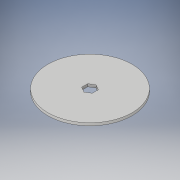
# Autodesk Inventor part: 4in Wheel Plate-ver1-1111-2019
Saved by Autodesk Inventor 2018 (Build 220112000, 112)
## iProperties
Created: 2020-01-18
Part Number: 4in Wheel Plate-ver1-1111-2019
Material: Generic
Document SubType Name: Modeling
Designer: JMHal
Density: 1 g/cm^3
Appearance: Default
Author: JMHal
Autodesk Inventor part; units mm, degrees
ref_plane "YZ Plane" through (0, 0, 0) normal (1, 0, 0) x (0, 1, 0)
ref_plane "XZ Plane" through (0, 0, 0) normal (0, 1, 0) x (-1, 0, 0)
ref_plane "XY Plane" through (0, 0, 0) normal (0, 0, 1) x (1, 0, 0)
sketch "Sketch1" plane through (0, 0, 0) normal (0, 1, 0) x (-1, 0, 0)
  circle A0 centre (0, 0) radius 50.8
  dimension "d0" = 101.6
  constraints: 1 centre point, 1 coincident
  measures "d0" diameter of A0
extrude "Extrusion1" add sketch "Sketch1" along normal blind 3.175
sketch "Sketch4" plane through (0, 3.175, 0) normal (0, 1, 0) x (1, 0, 0)
  line L0 (6.3399, 3.7001) -> (6.3743, -3.6405)
  line L1 (6.3743, -3.6405) -> (0.0344, -7.3406)
  line L2 (0.0344, -7.3406) -> (-6.3399, -3.7001)
  line L3 (-6.3399, -3.7001) -> (-6.3743, 3.6405)
  line L4 (-6.3743, 3.6405) -> (-0.0344, 7.3406)
  line L5 (-0.0344, 7.3406) -> (6.3399, 3.7001)
  point P0 (0, 0)
  point P1 (0, 0)
  dimension "d8" = 7.3406
  dimension "d9" = 0
  dimension "d10" = 0
  constraints: 12 end point, 13 other
  measures "d8" vertical distance of L2.end L3.end
  measures "d9" distance of point (0, 0) point (0, 0)
  measures "d10" distance of point (0, 0) point (0, 0)
extrude "Extrusion3" cut sketch "Sketch4" against normal blind 25.4
body "Solid1"
